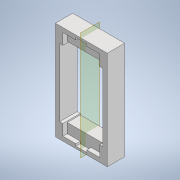
# Autodesk Inventor part: battery indicator case
Saved by Autodesk Inventor 2022 (Build 260153000, 153)
## iProperties
Created: 2021-10-19
Part Number: battery indicator case
Material: Generic
Document SubType Name: Modeling
Designer: tecware
Density: 1 g/cm^3
Appearance: Default
Author: tecware
Autodesk Inventor part; units mm, degrees
ref_plane "YZ Plane" through (0, 0, 0) normal (1, 0, 0) x (0, 1, 0)
ref_plane "XZ Plane" through (0, 0, 0) normal (0, 1, 0) x (-1, 0, 0)
ref_plane "XY Plane" through (0, 0, 0) normal (0, 0, 1) x (1, 0, 0)
sketch "Sketch1" plane through (0, 0, 0) normal (0, 0, 1) x (1, 0, 0)
  line L0 (-10, -15.65) -> (-10, 15.65) projected
  line L1 (-10, 15.65) -> (10, 15.65) projected
  line L2 (10, 15.65) -> (10, -15.65) projected
  line L3 (10, -15.65) -> (-10, -15.65) projected
  line L4 (1.5877, -12.1184) -> (1.5877, -10.9726) projected
  line L5 (5.119, -12.1184) -> (1.5877, -12.1184) projected
  line L6 (5.119, 11.1491) -> (5.119, -12.1184) projected
  line L7 (2.2936, 11.1491) -> (5.119, 11.1491) projected
  line L8 (2.2936, 12.739) -> (2.2936, 11.1491) projected
  line L9 (-2.2936, 12.739) -> (2.2936, 12.739) projected
  line L10 (-2.2936, 11.1491) -> (-2.2936, 12.739) projected
  line L11 (-5.119, 11.1491) -> (-2.2936, 11.1491) projected
  line L12 (-5.119, -12.1184) -> (-5.119, 11.1491) projected
  line L13 (-1.5877, -12.1184) -> (-5.119, -12.1184) projected
  line L14 (-1.5877, -10.9726) -> (-1.5877, -12.1184) projected
  line L15 (-4.1285, -10.9726) -> (-1.5877, -10.9726) projected
  line L16 (-4.1285, 10.0169) -> (-4.1285, -10.9726) projected
  line L17 (4.1285, 10.0169) -> (-4.1285, 10.0169) projected
  line L18 (4.1285, -10.9726) -> (4.1285, 10.0169) projected
  line L19 (1.5877, -10.9726) -> (4.1285, -10.9726) projected
  line L20 (2.9107, -1.4409) -> (2.9107, -4.3502) projected
  line L21 (-2.9107, -1.4409) -> (2.9107, -1.4409) projected
  line L22 (-2.9107, -4.3502) -> (-2.9107, -1.4409) projected
  line L23 (2.9107, -4.3502) -> (-2.9107, -4.3502) projected
  line L24 (2.9107, 7.9067) -> (2.9107, 4.9905) projected
  line L25 (-2.9107, 7.9067) -> (2.9107, 7.9067) projected
  line L26 (-2.9107, 4.9905) -> (-2.9107, 7.9067) projected
  line L27 (2.9107, 4.9905) -> (-2.9107, 4.9905) projected
  line L28 (2.9107, 3.2342) -> (2.9107, 0.4013) projected
  line L29 (-2.9107, 3.2342) -> (2.9107, 3.2342) projected
  line L30 (-2.9107, 0.4013) -> (-2.9107, 3.2342) projected
  line L31 (2.9107, 0.4013) -> (-2.9107, 0.4013) projected
  line L32 (2.9107, -6.1253) -> (2.9107, -8.9213) projected
  line L33 (-2.9107, -6.1253) -> (2.9107, -6.1253) projected
  line L34 (-2.9107, -8.9213) -> (-2.9107, -6.1253) projected
  line L35 (2.9107, -8.9213) -> (-2.9107, -8.9213) projected
  line L36 (-2.5, 20.75) -> (-8.5, 20.75) projected
  line L37 (-2.5, 21.75) -> (-2.5, 20.75) projected
  line L38 (2.5, 21.75) -> (-2.5, 21.75) projected
  line L39 (2.5, 20.75) -> (2.5, 21.75) projected
  line L40 (8.5, 20.75) -> (2.5, 20.75) projected
  line L41 (8.5, 15.65) -> (8.5, 20.75) projected
  line L42 (-8.5, 15.65) -> (8.5, 15.65) projected
  line L43 (-8.5, 20.75) -> (-8.5, 15.65) projected
  circle A0 centre (0, 18) radius 1.2 projected
  line L44 (-8.5, -15.65) -> (-8.5, -20.75) projected
  line L45 (8.5, -15.65) -> (-8.5, -15.65) projected
  line L46 (8.5, -20.75) -> (8.5, -15.65) projected
  line L47 (2.5, -20.75) -> (8.5, -20.75) projected
  line L48 (2.5, -21.75) -> (2.5, -20.75) projected
  line L49 (-2.5, -21.75) -> (2.5, -21.75) projected
  line L50 (-2.5, -20.75) -> (-2.5, -21.75) projected
  line L51 (-8.5, -20.75) -> (-2.5, -20.75) projected
  circle A1 centre (0, -18) radius 1.2 projected
  line L52 (12, 22.75) -> (-12, 22.75)
  line L53 (-12, 22.75) -> (-12, -22.75)
  line L54 (-12, -22.75) -> (12, -22.75)
  line L55 (12, -22.75) -> (12, 22.75)
  point P0 (0, 0)
  dimension "d0" = 2
  dimension "d1" = 2
  dimension "d2" = 2
  dimension "d3" = 2
  constraints: 8 end point, 2 parallel, 1 horizontal, 1 perpendicular
  measures "d0" distance between parallel lines of L2 L55
  measures "d1" distance between parallel lines of L0 L53
  measures "d2" distance between parallel lines of L36 L52
  measures "d3" distance between parallel lines of L54 L51
extrude "Extrusion1" add sketch "Sketch1" against normal blind 8 contours L55 L54 L53 L52
ref_plane "Work Plane1" through (0, -22.75, 0) normal (-1, 0, 0) x (0, 0, 1)
sketch "Sketch2" plane through (0, -22.75, 0) normal (-1, 0, 0) x (0, 0, 1)
  line L0 (0, 44.5) -> (-8, 44.5) projected
  line L1 (-8, 0) -> (-8, 45.5) projected
  line L2 (-2, 44.5) -> (-8, 44.5)
  line L3 (-8, 44.5) -> (-8, 39)
  line L4 (-8, 39) -> (-2, 39)
  line L5 (-2, 39) -> (-2, 44.5)
  line L6 (-8, 38.4) -> (-8, 7.1) projected
  line L7 (-8, 22.75) -> (6.4462, 22.75)
  line L8 (0, 1) -> (-8, 1)
  line L9 (-2, 1) -> (-8, 1)
  line L10 (-8, 1) -> (-8, 6.5)
  line L11 (-8, 6.5) -> (-2, 6.5)
  line L12 (-2, 6.5) -> (-2, 1)
  point P0 (0, 22.75)
  constraints: 20 end point, 6 symmetric about line, 3 point on line, 2 horizontal, 2 parallel, 1 midpoint, 1 perpendicular
extrude "Extrusion2" add sketch "Sketch2" along normal mid plane 24
sketch "Sketch3" plane through (0, 0, -8) normal (0, 0, -1) x (-1, 0, 0)
  line L0 (-12, 22.75) -> (-12, -22.75) projected
  line L1 (-12, 22.75) -> (12, 22.75)
  line L2 (12, 22.75) -> (12, -22.75)
  line L3 (12, -22.75) -> (-12, -22.75)
  line L4 (-12, -22.75) -> (-12, 22.75)
  line L5 (-6, -13) -> (6, -13)
  line L6 (6, -13) -> (6, 13)
  line L7 (6, 13) -> (-6, 13)
  line L8 (-6, 13) -> (-6, -13)
  point P0 (0, 0)
  constraints: 16 end point, 4 parallel, 2 horizontal, 2 perpendicular
extrude "Extrusion3" add sketch "Sketch3" along normal blind 2
chamfer "Chamfer1" distance 1 angle 45 4 edges at (0, 13, -10) (-6, 0, -10) (6, 0, -10) (0, -13, -10) measured on face at (-10, 4.3333, -10)
equation "\"d1\" = d0"
equation "\"d2\" = d1"
equation "\"d3\" = d1"
body "Solid1"
